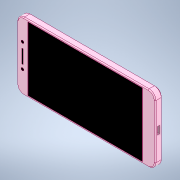
# Autodesk Inventor part: leeco
Saved by Autodesk Inventor 2020 (Build 240168000, 168)
## iProperties
Created: 2020-11-25
Part Number: leeco
Material: ABS Plastic
Document SubType Name: Modeling
Designer: Curtis
Density: 1.06 g/cm^3
Appearance: Smooth - White
Author: Curtis
Autodesk Inventor part; units mm, degrees
ref_plane "YZ Plane" through (0, 0, 0) normal (1, 0, 0) x (0, 1, 0)
ref_plane "XZ Plane" through (0, 0, 0) normal (0, 1, 0) x (-1, 0, 0)
ref_plane "XY Plane" through (0, 0, 0) normal (0, 0, 1) x (1, 0, 0)
sketch "Sketch1" plane through (0, 0, 0) normal (0, 1, 0) x (-1, 0, 0)
  line L0 (0, 0) -> (151.5, 0)
  line L1 (151.5, 0) -> (151.5, -74)
  line L2 (151.5, -74) -> (0, -74)
  line L3 (0, -74) -> (0, 0)
  dimension "d0" = 151.5
  dimension "d1" = 74
  constraints: 8 end point, 2 parallel, 1 horizontal, 1 perpendicular
  measures "d0" distance of L1.end L2.end
  measures "d1" distance of L0.end L1.end
extrude "Extrusion1" add sketch "Sketch1" along normal blind 7.7
sketch "Sketch2" plane through (0, 7.7, 0) normal (0, 1, 0) x (1, 0, 0)
  line L0 (-12.3, 29.65) -> (-27, 29.65)
  line L1 (-27, 29.65) -> (-27, 44.35)
  line L2 (-27, 44.35) -> (-12.3, 44.35)
  line L3 (-12.3, 44.35) -> (-12.3, 29.65)
  line L4 (-151.5, 0) -> (0, 0) projected
  line L5 (0, 74) -> (-151.5, 74) projected
  line L6 (0, 0) -> (0, 74) projected
  dimension "d4" = 14.7
  dimension "d5" = 14.7
  dimension "d6" = 44.35
  dimension "d7" = 44.35
  dimension "d8" = 12.3
  constraints: 8 end point, 2 parallel, 1 horizontal, 1 perpendicular
  measures "d4" distance of L1.end L2.end
  measures "d5" distance of L0.end L1.end
  measures "d6" distance between parallel lines of L4 L2
  measures "d7" distance between parallel lines of L5 L0
  measures "d8" distance between parallel lines of L6 L3
extrude "Extrusion2" add sketch "Sketch2" along normal blind 1
sketch "Sketch3" plane through (0, 0, 0) normal (0, -1, 0) x (1, 0, 0)
  line L0 (-12, -2) -> (-137.5, -2)
  line L1 (-137.5, -2) -> (-137.5, -72)
  line L2 (-137.5, -72) -> (-12, -72)
  line L3 (-12, -72) -> (-12, -2)
  line L4 (0, 0) -> (0, -74) projected
  line L5 (-151.5, -74) -> (-151.5, 0) projected
  line L6 (-151.5, 0) -> (0, 0) projected
  line L7 (0, -74) -> (-151.5, -74) projected
  dimension "d11" = 12
  dimension "d12" = 14
  dimension "d13" = 2
  dimension "d14" = 2
  constraints: 8 end point, 2 parallel, 1 horizontal, 1 perpendicular
  measures "d11" distance between parallel lines of L4 L3
  measures "d12" distance between parallel lines of L5 L1
  measures "d13" distance between parallel lines of L6 L0
  measures "d14" distance between parallel lines of L7 L2
extrude "Extrusion3" cut sketch "Sketch3" against normal blind 0.1 contours L3 L2 L1 L0
sketch "Sketch4" plane through (0, 0, 0) normal (0, -1, 0) x (1, 0, 0)
  circle A0 centre (-6, -24) radius 1.5
  circle A1 centre (-6, -50) radius 1.5
  line L0 (0, 0) -> (0, -74) projected
  line L1 (0, -74) -> (-151.5, -74) projected
  line L2 (-151.5, 0) -> (0, 0) projected
  line L3 (-6.65, -28.75) -> (-5.35, -28.75)
  line L4 (-5.35, -28.75) -> (-5.35, -43.75)
  line L5 (-5.35, -43.75) -> (-6.65, -43.75)
  line L6 (-6.65, -43.75) -> (-6.65, -28.75)
  line L7 (-12, -2) -> (-12, -72) projected
  dimension "d17" = 3
  dimension "d18" = 3
  dimension "d19" = 6
  dimension "d20" = 6
  dimension "d21" = 24
  dimension "d22" = 24
  dimension "d23" = 1.3
  dimension "d24" = 15
  dimension "d25" = 4.75
  dimension "d26" = 4.75
  dimension "d27" = 5.35
  dimension "d28" = 5.35
  constraints: 8 end point, 2 centre point, 2 parallel, 1 horizontal, 1 perpendicular
  measures "d17" diameter of A0
  measures "d18" diameter of A1
  measures "d19" distance from line of L0 A0.centre
  measures "d20" distance from line of L0 A1.centre
  measures "d21" distance from line of L1 A1.centre
  measures "d22" distance from line of L2 A0.centre
  measures "d23" distance of L3.start L3.end
  measures "d24" distance between parallel lines of L5 L3
  measures "d25" distance from line of A0.centre L3
  measures "d26" distance edge to line of A1 L5
  measures "d27" distance between parallel lines of L0 L4
  measures "d28" distance between parallel lines of L7 L6
extrude "Extrusion4" cut sketch "Sketch4" against normal blind 0.1
sketch "Sketch5" plane through (-151.5, 0, -74) normal (-1, 0, 0) x (0, 0, 1)
  line L0 (32.9, 2.7) -> (41.1, 2.7)
  line L1 (41.1, 2.7) -> (41.1, 5)
  line L2 (41.1, 5) -> (32.9, 5)
  line L3 (32.9, 5) -> (32.9, 2.7)
  line L4 (0, 0) -> (0, 7.7) projected
  line L5 (74, 0) -> (74, 7.7) projected
  line L6 (0, 7.7) -> (74, 7.7) projected
  line L7 (0, 0) -> (74, 0) projected
  dimension "d31" = 8.2
  dimension "d32" = 2.3
  dimension "d33" = 32.9
  dimension "d34" = 32.9
  dimension "d35" = 2.7
  dimension "d36" = 2.7
  constraints: 8 end point, 2 parallel, 1 horizontal, 1 perpendicular
  measures "d31" distance of L2.end L1.end
  measures "d32" distance of L1.end L0.end
  measures "d33" distance between parallel lines of L4 L3
  measures "d34" distance from line of L5 L0.end
  measures "d35" distance between parallel lines of L6 L2
  measures "d36" distance between parallel lines of L7 L0
extrude "Extrusion5" cut sketch "Sketch5" against normal blind 3.4 contours L3 L2 L1 L0
fillet "Fillet1" radius 7.5 4 edges at (0, 3.85, 0) (0, 3.85, -74) (-151.5, 3.85, 0) (-151.5, 3.85, -74)
chamfer "Chamfer1" distance 1 angle 45 16 edges at (0, 0, -37) (-2.1967, 0, -71.8033) (-75.75, 0, -74) (-149.3033, 0, -71.8033) (-151.5, 0, -37) (-149.3033, 0, -2.1967) (-75.75, 0, 0) (-2.1967, 0, -2.1967) (0, 7.7, -37) (-2.1967, 7.7, -71.8033) (-75.75, 7.7, -74) (-149.3033, 7.7, -71.8033) (-151.5, 7.7, -37) (-149.3033, 7.7, -2.1967) (-75.75, 7.7, 0) (-2.1967, 7.7, -2.1967)
sketch "Sketch6" plane through (0, 0, 0) normal (0, -1, 0) x (1, 0, 0)
  line L0 (-12, 0.5) -> (-7, 0.5)
  line L1 (0.5, -7) -> (0.5, -67)
  line L2 (-7, -74.5) -> (-12, -74.5)
  line L3 (-12, -74.5) -> (-12, 0.5)
  arc A0 (-7, -74.5) -> (0.5, -67) centre (-7, -67) ccw
  arc A1 (0.5, -7) -> (-7, 0.5) centre (-7, -7) ccw
  line L4 (-144, -74) -> (-7.5, -74) projected
  line L5 (-7.5, 0) -> (-144, 0) projected
  line L6 (0, -66.5) -> (0, -7.5) projected
  line L7 (-12, -2) -> (-12, -72) projected
  line L8 (-12, 3.5) -> (-4, 3.5)
  line L9 (3.5, -4) -> (3.5, -70)
  line L10 (-4, -77.5) -> (-12, -77.5)
  line L11 (-12, -77.5) -> (-12, 3.5)
  arc A2 (-4, -77.5) -> (3.5, -70) centre (-4, -70) ccw
  arc A3 (3.5, -4) -> (-4, 3.5) centre (-4, -4) ccw
  circle A4 centre (-6, -50) radius 1.5 projected
  circle A5 centre (-6, -50) radius 2.5
  circle A6 centre (-6, -24) radius 1.5 projected
  circle A7 centre (-6, -24) radius 2.5
  line L12 (-137.5, 0.5) -> (-144.5, 0.5)
  line L13 (-152, -7) -> (-152, -67)
  line L14 (-144.5, -74.5) -> (-137.5, -74.5)
  line L15 (-137.5, -74.5) -> (-137.5, 0.5)
  line L16 (-151.5, -7.5) -> (-151.5, -66.5) projected
  line L17 (-137.5, -72) -> (-137.5, -2) projected
  arc A8 (-152, -67) -> (-144.5, -74.5) centre (-144.5, -67) ccw
  arc A9 (-144.5, 0.5) -> (-152, -7) centre (-144.5, -7) ccw
  line L18 (-137.5, 3.5) -> (-147.5, 3.5)
  line L19 (-155, -4) -> (-155, -70)
  line L20 (-147.5, -77.5) -> (-137.5, -77.5)
  line L21 (-137.5, -77.5) -> (-137.5, 3.5)
  arc A10 (-155, -70) -> (-147.5, -77.5) centre (-147.5, -70) ccw
  arc A11 (-147.5, 3.5) -> (-155, -4) centre (-147.5, -4) ccw
  point P0 (0, 0)
  dimension "d43" = 7.5
  dimension "d44" = 0.5
  dimension "d45" = 0.5
  dimension "d46" = 0.5
  dimension "d47" = 0
  dimension "d48" = 0
  dimension "d49" = 3
  dimension "d50" = 3
  dimension "d51" = 3
  dimension "d52" = 7.5
  dimension "d53" = 5
  dimension "d54" = 5
  dimension "d55" = 0.5
  dimension "d56" = 0.5
  dimension "d57" = 0.5
  dimension "d58" = 0
  dimension "d59" = 7.5
  dimension "d60" = 7.5
  dimension "d61" = 3
  dimension "d62" = 3
  dimension "d63" = 3
  dimension "d64" = 0
  constraints: 32 end point, 16 point on circle, 16 tangent, 10 centre point, 8 parallel, 4 equal radius, 4 horizontal, 4 perpendicular, 2 coincident
  measures "d43" radius of A0
  measures "d44" distance between parallel lines of L4 L2
  measures "d45" distance between parallel lines of L5 L0
  measures "d46" distance between parallel lines of L6 L1
  measures "d47" distance between parallel lines of L7 L3
  measures "d48" distance between parallel lines of L7 L11
  measures "d49" distance between parallel lines of L0 L8
  measures "d50" distance between parallel lines of L2 L10
  measures "d51" distance between parallel lines of L1 L9
  measures "d52" radius of A2
  measures "d53" diameter of A5
  measures "d54" diameter of A7
  measures "d55" distance between parallel lines of L16 L13
  measures "d56" distance between parallel lines of L4 L14
  measures "d57" distance between parallel lines of L5 L12
  measures "d58" distance between parallel lines of L17 L15
  measures "d59" radius of A8
  measures "d60" radius of A10
  measures "d61" distance between parallel lines of L13 L19
  measures "d62" distance between parallel lines of L14 L20
  measures "d63" distance between parallel lines of L12 L18
  measures "d64" distance between parallel lines of L17 L21
extrude "Extrusion6" add sketch "Sketch6" along normal blind 3 separate body contours L11 L8 A3 L9 A2 L10 L2 A0 L1 A1 L0 | L0 A1 L1 A0 L2 L3 | L15 L14 A8 L13 A9 L12 | L12 A9 L13 A8 L14 L21 L20 A10 L19 A11 L18
extrude "Extrusion7" add sketch "Sketch6" against normal blind 8.5 contours L11 L8 A3 L9 A2 L10 L2 A0 L1 A1 L0 | L12 A9 L13 A8 L14 L21 L20 A10 L19 A11 L18 bodies 2
sketch "Sketch7" plane through (0, 8.5, 0) normal (0, 1, 0) x (1, 0, 0)
  line L0 (-4, -3.5) -> (-147.5, -3.5)
  line L1 (-155, 4) -> (-155, 70)
  line L2 (-147.5, 77.5) -> (-4, 77.5)
  line L3 (3.5, 70) -> (3.5, 4)
  line L4 (-147.5, -3.5) -> (-137.5, -3.5) projected
  line L5 (3.5, 4) -> (3.5, 70) projected
  line L6 (-4, 77.5) -> (-12, 77.5) projected
  line L7 (-155, 70) -> (-155, 4) projected
  arc A0 (-4, -3.5) -> (3.5, 4) centre (-4, 4) ccw
  arc A1 (-155, 4) -> (-147.5, -3.5) centre (-147.5, 4) ccw
  arc A2 (-147.5, 77.5) -> (-155, 70) centre (-147.5, 70) ccw
  arc A3 (3.5, 70) -> (-4, 77.5) centre (-4, 70) ccw
  point P0 (0, 0)
  dimension "d69" = 0
  dimension "d70" = 0
  dimension "d71" = 0
  dimension "d72" = 0
  dimension "d73" = 7.5
  constraints: 8 end point, 8 point on circle, 8 tangent, 4 centre point, 3 equal radius, 2 parallel, 1 horizontal, 1 perpendicular
  measures "d69" distance between parallel lines of L4 L0
  measures "d70" distance between parallel lines of L5 L3
  measures "d71" distance between parallel lines of L6 L2
  measures "d72" distance between parallel lines of L7 L1
  measures "d73" radius of A0
extrude "Extrusion8" add sketch "Sketch7" along normal blind 39 bodies 2
sketch "Sketch8" plane through (-137.5, -3, -77.5) normal (0, 0, -1) x (-1, 0, 0)
  line L0 (-91.25, 50.5) -> (-31.25, 50.5)
  line L1 (-31.25, 50.5) -> (-31.25, 25.5)
  line L2 (-31.25, 25.5) -> (-91.25, 25.5)
  line L3 (-91.25, 25.5) -> (-91.25, 50.5)
  line L4 (-133.5, 50.5) -> (10, 50.5) projected
  line L5 (17.5, 50.5) -> (17.5, 0) projected
  line L6 (-91.25, 50.5) -> (-141, 27.0493)
  line L7 (-141, 50.5) -> (-141, 0) projected
  line L8 (-31.25, 50.5) -> (17.5, 25.0356)
  line L9 (-141, 27.0493) -> (-141, 50.5)
  line L10 (-91.25, 50.5) -> (-141, 50.5)
  line L11 (-31.25, 50.5) -> (17.5, 50.5)
  line L12 (17.5, 25.0356) -> (17.5, 50.5)
  point P0 (-137.5, 3)
  point P1 (-31.25, 50.5)
  dimension "d76" = 60
  dimension "d77" = 25
  dimension "d78" = 0
  dimension "d79" = 48.75
  dimension "d80" = 55
  dimension "d81" = 55
  constraints: 20 end point, 2 collinear, 2 parallel, 2 point on line, 1 horizontal, 1 perpendicular
  measures "d76" distance of L0.start L0.end
  measures "d77" distance of L0.end L1.end
  measures "d78" distance between parallel lines of L4 L0
  measures "d79" distance between parallel lines of L5 L1
  measures "d80" distance of L0.start L6.end
  measures "d81" distance of L0.end L8.end
extrude "Extrusion9" cut sketch "Sketch8" against normal blind 105.25 contours L4 L11 L5 L8 | L6 L7 L10 L4 bodies 2
sketch "Sketch9" plane through (-155, -3, -70) normal (-1, 0, 0) x (0, 0, 1)
  line L0 (-4.5, 2.5) -> (70.5, 2.5)
  line L1 (70.5, 2.5) -> (70.5, 11.2)
  line L2 (70.5, 11.2) -> (-4.5, 11.2)
  line L3 (-4.5, 11.2) -> (-4.5, 2.5)
  line L4 (-4, 9.7) -> (-4, 4) projected
  line L5 (3.5, 3) -> (62.5, 3) projected
  line L6 (62.5, 10.7) -> (3.5, 10.7) projected
  line L7 (70, 4) -> (70, 9.7) projected
  point P0 (70, 3)
  dimension "d84" = 0.5
  dimension "d85" = 0.5
  dimension "d86" = 0.5
  dimension "d87" = 0.5
  constraints: 8 end point, 2 parallel, 1 horizontal, 1 perpendicular
  measures "d84" distance between parallel lines of L4 L3
  measures "d85" distance between parallel lines of L5 L0
  measures "d86" distance between parallel lines of L6 L2
  measures "d87" distance between parallel lines of L7 L1
extrude "Extrusion10" cut sketch "Sketch9" against normal blind 63 bodies 2
sketch "Sketch10" plane through (-155, 22.0356, -70) normal (-1, 0, 0) x (0, 0, 1)
  line L0 (2.5, -14.3356) -> (63.5, -14.3356)
  line L1 (63.5, -14.3356) -> (63.5, -4.3356)
  line L2 (63.5, -4.3356) -> (2.5, -4.3356)
  line L3 (2.5, -4.3356) -> (2.5, -14.3356)
  line L4 (62.5, -14.3356) -> (3.5, -14.3356) projected
  line L5 (70, -21.0356) -> (70, -15.3356) projected
  point P0 (70, -22.0356)
  dimension "d90" = 61
  dimension "d91" = 10
  dimension "d92" = 0
  dimension "d93" = 6.5
  constraints: 8 end point, 2 parallel, 1 horizontal, 1 perpendicular
  measures "d90" distance of L1.end L2.end
  measures "d91" distance of L2.end L0.start
  measures "d92" distance between parallel lines of L4 L0
  measures "d93" distance between parallel lines of L5 L1
extrude "Extrusion11" cut sketch "Sketch10" against normal blind 213.75 bodies 2
sketch "Sketch11" plane through (-153.5, 8.2, -74.5) normal (0, -1, 0) x (1, 0, 0)
  line L0 (9, 0) -> (0, 0)
  line L1 (-1.5, 4.5) -> (-1.5, 7) projected
  line L2 (1.5167, 7) -> (-1.5, 7)
  line L3 (-1.5, 4.5) -> (-1.5, 7)
  line L4 (153.9833, 7) -> (1.5167, 7) projected
  line L5 (9, 0) -> (16, 0) projected
  arc A0 (-1.5, 4.5) -> (0, 0) centre (6, 4.5) ccw projected
  arc A1 (-1.5, 4.5) -> (0, 0) centre (6, 4.5) ccw
  arc A2 (1.5167, 7) -> (9, 0) centre (9, 7.5) ccw
  arc A3 (1.5167, 7) -> (9, 0) centre (9, 7.5) ccw projected
  point P0 (153.5, 74.5)
  constraints: 6 end point, 4 point on circle, 2 centre point, 2 concentric, 2 horizontal, 1 collinear
extrude "Extrusion12" cut sketch "Sketch11" against normal up to surface (0.3 mm away) bodies 2
sketch "Sketch12" plane through (-153.5, 8.2, 0.5) normal (0, -1, 0) x (1, 0, 0)
  line L0 (-1.5, -7) -> (-1.5, -4.5) projected
  line L1 (-1.5, -7) -> (-1.5, -4.5)
  line L2 (1.5167, -7) -> (-1.5, -7)
  line L3 (0, 0) -> (9, 0) projected
  line L4 (0, 0) -> (9, 0)
  arc A0 (9, 0) -> (1.5167, -7) centre (9, -7.5) ccw
  arc A1 (9, 0) -> (1.5167, -7) centre (9, -7.5) ccw projected
  arc A2 (0, 0) -> (-1.5, -4.5) centre (6, -4.5) ccw
  arc A3 (0, 0) -> (-1.5, -4.5) centre (6, -4.5) ccw projected
  point P0 (153.5, -0.5)
  constraints: 6 end point, 4 point on circle, 2 centre point, 2 concentric, 1 collinear, 1 horizontal, 1 vertical
extrude "Extrusion13" cut sketch "Sketch12" against normal up to surface (0.3 mm away) bodies 2
sketch "Sketch13" plane through (-155, 8.5, -4) normal (-1, 0, 0) x (0, 0, 1)
  line L0 (-70.5, 9.2) -> (4.5, 9.2)
  line L1 (4.5, 9.2) -> (4.5, 36)
  line L2 (4.5, 36) -> (-70.5, 36)
  line L3 (-70.5, 36) -> (-70.5, 9.2)
  line L4 (-73.5, 17.4532) -> (-73.5, 39) projected
  line L5 (7.5, 39) -> (7.5, 17.4532) projected
  line L6 (-73.5, 39) -> (7.5, 39) projected
  line L7 (-63.5, 9.2) -> (-2.5, 9.2) projected
  point P0 (4, -8.5)
  dimension "d100" = 3
  dimension "d101" = 3
  dimension "d102" = 3
  dimension "d103" = 0
  constraints: 8 end point, 2 parallel, 1 horizontal, 1 perpendicular
  measures "d100" distance between parallel lines of L4 L3
  measures "d101" distance between parallel lines of L5 L1
  measures "d102" distance between parallel lines of L6 L2
  measures "d103" distance between parallel lines of L7 L0
extrude "Extrusion14" cut sketch "Sketch13" against normal blind 219.75 bodies 2
body "Solid1"
body "Solid2"
